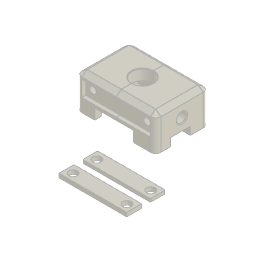
Obal_kamera (Autodesk Fusion 360 design; units mm, degrees)
part number: 2026-04-14-16-43-13-347
part number: 2026-04-14-16-45-35-834
Autodesk Fusion 360 part; units mm, degrees
sketch "Sketch1" plane through (0, 0, 0) normal (0, 0, 1) x (1, 0, 0) in component "kamera_obal"
  line L0 (-15, 10) -> (15, 10)
  line L1 (15, 10) -> (15, -10)
  line L2 (15, -10) -> (-15, -10)
  line L3 (-15, -10) -> (-15, 10)
  line L4 (-15, 10) -> (15, -10) construction
  line L5 (15, 10) -> (-15, -10) construction
  dimension "d1" = 20
  dimension "d2" = 30
  constraint horizontal L0
  constraint perpendicular L0 L1
  constraint parallel L0 L2
  constraint parallel L1 L3
  constraint coincident L4 origin
  constraint coincident L5 origin
  measures "d1" distance of L0.end L1.end
  measures "d2" distance of L1.end L2.end
extrude "Extrude1" add sketch "Sketch1" along normal blind 11 makes body 1 in component "kamera_obal"
sketch "Sketch4" plane through (0, 0, 11) normal (0, 0, 1) x (-1, 0, 0) in component "kamera_obal"
  line L0 (15, 10) -> (-15, 10)
  line L1 (-15, 10) -> (-15, -10)
  line L2 (-15, -10) -> (15, -10)
  line L3 (15, -10) -> (15, 10)
  circle A0 centre (0, 0) radius 4
  circle A1 centre (0, 0) radius 5.5
  dimension "d11" = 8
  dimension "d12" = 1.5
  constraint coincident A0.centre A1.centre
  measures "d11" diameter of A0
sketch "Sketch5" plane through (0, 0, 0) normal (0, 0, -1) x (1, 0, 0) in component "kamera_obal"
  line L0 (15, 10) -> (-15, 10)
  line L1 (-15, 10) -> (-15, -10)
  line L2 (-15, -10) -> (15, -10)
  line L3 (15, -10) -> (15, 10)
  line L4 (-4, 4) -> (4, 4) construction
  line L5 (4, 4) -> (4, -4) construction
  line L6 (4, -4) -> (-4, -4) construction
  line L7 (-4, -4) -> (-4, 4) construction
  line L8 (-4, 4) -> (4, -4) construction
  line L9 (4, 4) -> (-4, -4) construction
  line L10 (-4, 4) -> (-4, 7.4) construction
  line L11 (-4, 4) -> (-8, 4) construction
  line L12 (-4, -4) -> (-4, -6.3) construction
  line L13 (4, -4) -> (6.6, -4) construction
  line L14 (-4, -4) -> (-7.2, -4) construction
  line L15 (-7.2, -4) -> (-4, -4) construction
  line L16 (-4, -4) -> (-4, -6.3) construction
  line L17 (-4, -6.3) -> (-7.2, -6.3) construction
  line L18 (-7.2, -6.3) -> (-7.2, -4) construction
  line L19 (-4, -6.3) -> (6.5, -6.3) construction
  line L20 (6.6, -4) -> (4, -4) construction
  line L21 (4, -4) -> (4, -6.3) construction
  line L22 (4, -6.3) -> (6.6, -6.3) construction
  line L23 (6.6, -6.3) -> (6.6, -4) construction
  line L24 (-4, 7.4) -> (-8, 7.4) construction
  line L25 (-8, 7.4) -> (-8, 4) construction
  line L26 (-8, 4) -> (-4, 4) construction
  line L27 (-4, 4) -> (-4, 7.4) construction
  line L28 (6.6, -6.3) -> (-8.1, -6.3) construction
  line L29 (-8.1, -6.3) -> (-7.2, -6.3) construction
  line L30 (-7.2, -6.3) -> (6.1, -6.3) construction
  line L31 (6.1, -6.3) -> (6.6, -6.3) construction
  line L32 (6.6, -6.3) -> (-8.1, -6.3)
  line L33 (-8.1, -6.3) -> (-8.1, 7.5)
  line L34 (-8.1, 7.5) -> (6.6, 7.5)
  line L35 (6.6, 7.5) -> (6.6, -6.3)
  dimension "d13" = 8
  dimension "d14" = 8
  dimension "d15" = 4
  dimension "d17" = 2.3
  dimension "d18" = 2.6
  dimension "d143" = 4.1
  dimension "d144" = 3.5
  constraint horizontal L4
  constraint perpendicular L4 L5
  constraint parallel L4 L6
  constraint parallel L5 L7
  constraint coincident L8 origin
  constraint coincident L9 origin
  constraint perpendicular L4 L10
  constraint perpendicular L7 L11
  constraint perpendicular L6 L12
  constraint perpendicular L5 L13
  constraint perpendicular L12 L14
  constraint horizontal L15
  constraint vertical L16
  constraint horizontal L17
  constraint vertical L18
  constraint perpendicular L12 L19
  constraint horizontal L20
  constraint vertical L21
  constraint horizontal L22
  constraint vertical L23
  constraint coincident L19 L21.end
  constraint horizontal L24
  constraint vertical L25
  constraint horizontal L26
  constraint vertical L27
  constraint horizontal L28
  constraint horizontal L30
  constraint perpendicular L32 L33
  constraint parallel L32 L34
  constraint parallel L33 L35
  measures "d13" distance of L4.end L5.end
  measures "d14" distance of L5.end L6.end
  measures "d15" distance of L4.start L11.end
  measures "d17" distance of L6.end L12.end
  measures "d18" distance of L5.end L13.end
  measures "d143" distance of L7 L33
  measures "d144" distance of L4 L34
extrude "Extrude3" cut sketch "Sketch5" against normal blind 9 contours L32 L33 L34 L35 bodies 1 in component "kamera_obal"
extrude "Extrude4" add sketch "Sketch4" along normal blind 2.2 contours A1 bodies 1 in component "kamera_obal"
extrude "Extrude5" cut 1 faces at (-0.9485, -1.8197, 11) along direction (0, 0, -1) blind 2 on bodies 1 bodies 1 in component "kamera_obal"
extrude "Extrude25" add 1 faces at (-11.8333, 0, 11) along direction (0, 0, 1) blind 2.2 on bodies 1 bodies 1 in component "kamera_obal"
sketch "Sketch7" plane through (0, 10, 0) normal (0, 1, 0) x (-1, 0, 0) in component "kamera_obal"
  line L0 (-15, 13.2) -> (-15, 0)
  line L1 (-15, 0) -> (15, 0)
  line L2 (-6.6, 0) -> (-6.6, 9) construction
  line L3 (8.1, 0) -> (8.1, 9) construction
  line L4 (15, 0) -> (15, 13.2) construction
  line L5 (-6.6, 9) -> (8.1, 9) construction
  line L6 (-6.6, 0) -> (-6.6, 4)
  line L7 (-6.6, 4) -> (8.1, 4)
  line L8 (8.1, 4) -> (8.1, 0)
  line L9 (0, 4) -> (0, 5) construction
  line L10 (-13, 5) -> (13, 5) construction
  line L11 (-13, 5) -> (13, 5)
  line L12 (13, 5) -> (13, 11)
  line L13 (13, 11) -> (-13, 11)
  line L14 (-13, 11) -> (-13, 5)
  line L15 (15, 13.2) -> (-15, 13.2)
  point P0 (0, 5.5)
  dimension "d57" = 6
  dimension "d145" = 4
  dimension "d146" = 26
  dimension "d147" = 1
  constraint perpendicular L1 L6
  constraint perpendicular L2 L7
  constraint coincident L1 L3.start
  constraint perpendicular L1 L8
  constraint midpoint L9.end L10
  constraint horizontal L11
  constraint vertical L12
  constraint horizontal L13
  constraint vertical L14
  constraint coincident L3 L7.end
  constraint coincident L7 L9.start
  constraint horizontal L7.end L8.start
  constraint coincident L7.end L8.start
  constraint vertical L2.start L6.end
  constraint midpoint L9.end L11
  constraint vertical L9
  constraint vertical origin L9.start
  measures "d57" distance of L10.start L13.end
  measures "d145" distance of L7.end L3.start
  measures "d146" distance of L12.end L13.end
  measures "d147" distance of L7 L11
extrude "Extrude23" cut sketch "Sketch7" against normal blind 7 contours L1 L6 L7 L8 bodies 1 in component "kamera_obal"
extrude "Extrude8" cut sketch "Sketch7" against normal blind 1.5 contours L11 L12 L13 L14 bodies 1 in component "kamera_obal"
sketch "Sketch11" plane through (0, -10, 0) normal (0, -1, 0) x (1, 0, 0) in component "kamera_obal"
  line L0 (-15, 0) -> (15, 0)
  line L1 (15, 0) -> (15, 13.2)
  line L2 (-15, 13.2) -> (-15, 0)
  line L3 (13, 11) -> (-13, 11)
  line L4 (13, 5) -> (13, 11)
  line L5 (-13, 11) -> (-13, 5)
  line L6 (-13, 5) -> (13, 5)
  line L7 (6.6, 0) -> (6.6, 4)
  line L8 (6.6, 4) -> (-8.1, 4)
  line L9 (-8.1, 4) -> (-8.1, 0)
  line L10 (15, 13.2) -> (-15, 13.2)
extrude "Extrude24" cut sketch "Sketch11" against normal blind 7 contours L0 L7 L8 L9 bodies 1 in component "kamera_obal"
extrude "Extrude10" cut sketch "Sketch11" against normal blind 1.5 contours L3 L4 L5 L6 bodies 1 in component "kamera_obal"
sketch "Sketch9" plane through (15, 0, 0) normal (1, 0, 0) x (0, 1, 0) in component "kamera_obal"
  line L0 (-10, 0) -> (10, 0)
  line L1 (10, 0) -> (10, 13.2)
  line L2 (-10, 13.2) -> (-10, 0)
  circle A0 centre (0, 7.3632) radius 1.85
  line L3 (-10, 0) -> (-4.4, 0) construction
  line L4 (10, 0) -> (3.1, 0) construction
  line L5 (-4.4, 0) -> (-4.4, 3) construction
  line L6 (-4.4, 3) -> (3.1, 3)
  line L7 (3.1, 3) -> (3.1, 0)
  line L8 (3.1, 0) -> (-4.4, 0)
  line L9 (-4.4, 0) -> (-4.4, 3)
  line L10 (-10, 1.5263) -> (10, 13.2) construction
  line L11 (-10, 0) -> (10, 0)
  line L12 (10, 0) -> (10, 4)
  line L13 (10, 4) -> (6.3, 4)
  line L14 (6.3, 4) -> (6.3, 9)
  line L15 (6.3, 9) -> (-7.5, 9)
  line L16 (-7.5, 9) -> (-7.5, 4)
  line L17 (-7.5, 4) -> (-10, 4)
  line L18 (-10, 4) -> (-10, 0)
  line L19 (-7.5, 4) -> (-7.5, 0) construction
  line L20 (6.3, 4) -> (6.3, 0) construction
  line L21 (10, 13.2) -> (-10, 13.2)
  dimension "d41" = 3.7
  dimension "d66" = 3
  dimension "d154" = 3.1
  dimension "d155" = 4
  dimension "d156" = 3.2
  constraint coincident L0.start L2.end
  constraint perpendicular L2 L3
  constraint coincident L0.end L1.start
  constraint perpendicular L1 L4
  constraint perpendicular L3 L5
  constraint horizontal L6
  constraint vertical L7
  constraint horizontal L8
  constraint vertical L9
  constraint coincident L2 L10.start
  constraint coincident L1.end L10.end
  constraint midpoint A0.centre L10
  constraint coincident L16.end L17.start
  constraint coincident L11 L19.end
  constraint coincident L13.end L14.start
  constraint perpendicular L4 L20
  measures "d41" diameter of A0
  measures "d66" distance of L3.end L5.end
  measures "d154" distance of L5 L19
  measures "d155" distance of L13.end L20.end
  measures "d156" distance of L7 L20
sketch "Sketch10" plane through (-15, 0, 0) normal (-1, 0, 0) x (0, -1, 0) in component "kamera_obal"
  line L0 (-10, 0) -> (10, 0)
  line L1 (10, 0) -> (10, 13.2)
  line L2 (-10, 13.2) -> (-10, 0)
  circle A0 centre (0, 7.3632) radius 1.85
  line L3 (3, 3) -> (7.5, 3)
  line L4 (7.5, 3) -> (7.5, 0)
  line L5 (-10, 0) -> (10, 0)
  line L6 (10, 0) -> (10, 4)
  line L7 (10, 4) -> (7.5, 4)
  line L8 (7.5, 4) -> (7.5, 9)
  line L9 (7.5, 9) -> (-6.3, 9)
  line L10 (-6.3, 9) -> (-6.3, 4)
  line L11 (-6.3, 4) -> (-10, 4)
  line L12 (-10, 4) -> (-10, 0)
  line L13 (3, 3) -> (3, 0)
  line L14 (10, 13.2) -> (-10, 13.2)
  dimension "d152" = 4.5
  dimension "d153" = 3
  constraint horizontal L3
  constraint vertical L4
  constraint horizontal L0.end L4.end
  constraint coincident L0 L13.end
  constraint perpendicular L0 L13
  constraint vertical L3.end L7.end
  measures "d152" distance of L3.start L3.end
  measures "d153" distance of L3.end L4.end
extrude "Extrude12" cut sketch "Sketch9" against normal blind 4.7 contours A0 L15 | A0 L15 bodies 1 in component "kamera_obal"
extrude "Extrude13" cut sketch "Sketch9" against normal blind 15 contours L0 L6 L7 L8 L9 L11 bodies 1 in component "kamera_obal"
extrude "Extrude14" cut sketch "Sketch10" against normal blind 4.7 contours A0 L9 | A0 L9 bodies 1 in component "kamera_obal"
extrude "Extrude15" cut sketch "Sketch10" against normal blind 15 contours L0 L3 L4 L5 L13 bodies 1 in component "kamera_obal"
ref_plane "WorkPlane2" through (0, 0, 0) normal (1, 0, 0) x (0, 1, 0) in component "kamera_obal"
ref_plane "WorkPlane5" through (0, 8.5, 5.5) normal (0, 1, 0) x (-1, 0, 0) in component "kamera_obal"
sketch "Sketch14" plane through (0, 8.5, 0) normal (0, 1, 0) x (1, 0, 0) in component "kamera_obal"
  line L0 (6.6, -4) -> (6.6, -9)
  line L1 (-8.1, -4) -> (-8.1, -9)
  line L2 (13, -11) -> (-13, -11) construction
  line L3 (13, -5) -> (13, -11) construction
  line L4 (-13, -5) -> (13, -5) construction
  line L5 (-13, -11) -> (-13, -5) construction
  line L6 (6.6, -5) -> (6.6, -5.8) construction
  line L7 (6.6, -5.8) -> (12.5, -5.8) construction
  line L8 (8.05, -9.2) -> (8.05, -10) construction
  line L9 (8.05, -9.2) -> (13.95, -9.2) construction
  line L10 (8.05, -9.2) -> (9.05, -9.2) construction
  line L11 (9.05, -9.2) -> (11.45, -9.2) construction
  line L12 (11.45, -9.2) -> (11.45, -6.8) construction
  line L13 (11.45, -6.8) -> (9.05, -6.8) construction
  line L14 (9.05, -6.8) -> (9.05, -9.2) construction
  line L15 (11.45, -6.8) -> (9.05, -9.2) construction
  circle A0 centre (10.25, -8) radius 1.25
  line L16 (-8.1, -5) -> (-8.1, -5.8) construction
  line L17 (-8.1, -9) -> (-8.1, -9.2) construction
  line L18 (-9.05, -9.2) -> (-11.45, -9.2) construction
  line L19 (-9.05, -9.2) -> (-9.05, -6.8) construction
  line L20 (-9.05, -6.8) -> (-11.45, -9.2) construction
  circle A1 centre (-10.25, -8) radius 1.25
  line L21 (-8.1, -3) -> (-8.1, 0)
  dimension "d96" = 0.8
  dimension "d97" = 5.9
  dimension "d99" = 0.8
  dimension "d100" = 5.9
  dimension "d101" = 1
  dimension "d102" = 2.4
  dimension "d103" = 2.4
  dimension "d104" = 2.5
  dimension "d108" = 2.4
  dimension "d109" = 2.4
  dimension "d110" = 2.5
  dimension "d161" = 1.8
  dimension "d164" = 1.8
  dimension "d166" = 2.75
  dimension "d169" = 2.75
  constraint coincident L4 L6.start
  constraint coincident L0 L6.start
  constraint perpendicular L4 L6
  constraint perpendicular L3 L7
  constraint perpendicular L2 L8
  constraint perpendicular L3 L9
  constraint perpendicular L8 L10
  constraint horizontal L11
  constraint vertical L12
  constraint horizontal L13
  constraint vertical L14
  constraint midpoint L15 A0.centre
  constraint coincident L4 L16.start
  constraint coincident L1 L16.start
  constraint perpendicular L4 L16
  constraint coincident L1.end L17.start
  constraint perpendicular L2 L17
  constraint perpendicular L18 L19
  constraint midpoint L20 A1.centre
  constraint parallel L2 L18
  measures "d96" distance of L6.start L6.end
  measures "d97" distance of L6.end L7.end
  measures "d99" distance of L8.start L8.end
  measures "d100" distance of L8.start L9.end
  measures "d101" distance of L8.start L10.end
  measures "d102" distance of L10.end L13.end
  measures "d103" distance of L10.end L11.end
  measures "d104" diameter of A0
  measures "d108" distance of L18.start L18.end
  measures "d109" distance of L18.start L19.end
  measures "d110" diameter of A1
  measures "d161" distance of L4 L13
  measures "d164" distance of L2 L18
  measures "d166" distance of L5 A1.centre
  measures "d169" distance of L3 A0.centre
extrude "Extrude19" cut sketch "Sketch14" against normal blind 5 contours A0 bodies 1 in component "kamera_obal"
extrude "Extrude20" cut sketch "Sketch14" against normal blind 5 contours A1 bodies 1 in component "kamera_obal"
ref_plane "WorkPlane6" through (0, -8.5, 8) normal (0, -1, 0) x (0, 0, -1) in component "kamera_obal"
sketch "Sketch15" plane through (0, -8.5, 0) normal (0, -1, 0) x (-1, 0, 0) in component "kamera_obal"
  circle A0 centre (10.25, -8) radius 1.25
  circle A1 centre (-10.25, -8) radius 1.25
extrude "Extrude21" cut sketch "Sketch15" against normal blind 5 contours A0 bodies 1 in component "kamera_obal"
extrude "Extrude22" cut sketch "Sketch15" against normal blind 5 contours A1 bodies 1 in component "kamera_obal"
fillet "Fillet1" radius 2 4 edges at (15, 10, 5.5) (-15, 10, 5.5) (-15, -10, 5.5) (15, -10, 5.5) on bodies 1 in component "kamera_obal"
chamfer "Chamfer2" distance 2 distance2 1.5 8 edges at (0, -10, 13.2) (14.4142, -9.4142, 13.2) (15, 0, 13.2) (14.4142, 9.4142, 13.2) (0, 10, 13.2) (-14.4142, 9.4142, 13.2) (-15, 0, 13.2) (-14.4142, -9.4142, 13.2) measured on face at (-11.3333, 0, 13.2) measured on face at (13.0955, -9.9977, 8.8) measured on face at (-11.3333, 0, 13.2) measured on face at (14.7321, 9.0002, 8.8) measured on face at (-11.3333, 0, 13.2) measured on face at (-14.9977, 8.0955, 4.4) measured on face at (-11.3333, 0, 13.2) measured on face at (-13.0955, -9.9977, 4.4) on bodies 1 in component "kamera_obal"
sketch "Sketch2" plane through (0, 0, 0) normal (0, 0, 1) x (1, 0, 0)
  line L0 (4, -21) -> (29.7, -21)
  line L1 (29.7, -21) -> (29.7, -26.7)
  line L2 (29.7, -26.7) -> (4, -26.7)
  line L3 (4, -26.7) -> (4, -21)
  dimension "d124" = 5.7
  dimension "d125" = 25.7
  constraint horizontal L0
  constraint vertical L1
  constraint horizontal L2
  constraint vertical L3
  measures "d124" distance of L0.start L2.end
  measures "d125" distance of L0.start L0.end
extrude "Extrude1'" add sketch "Sketch2" along normal blind 1.5 separate body makes body 2
sketch "Sketch4 (2)" plane through (0, 0, 1.5) normal (0, 0, 1) x (-1, 0, 0)
  line L0 (-4, 26.7) -> (-29.7, 26.7)
  line L1 (-29.7, 26.7) -> (-29.7, 21)
  line L2 (-29.7, 21) -> (-4, 21)
  line L3 (-4, 21) -> (-4, 26.7)
  line L4 (-7.8185, 26.8595) -> (-7.8654, 25.2102) construction
  line L5 (-7.8654, 25.2102) -> (-5.4664, 25.142) construction
  line L6 (-7.8654, 25.2102) -> (-7.9336, 22.8112) construction
  line L7 (-5.4664, 25.142) -> (-7.9336, 22.8112) construction
  circle A0 centre (-6.7, 23.9766) radius 1.6
  line L8 (-25.793, 26.7352) -> (-25.7977, 25.0852) construction
  line L9 (-25.7977, 25.0852) -> (-25.8023, 22.6853) construction
  line L10 (-25.7977, 25.0852) -> (-28.1977, 25.0898) construction
  line L11 (-25.8023, 22.6853) -> (-28.1977, 25.0898) construction
  circle A1 centre (-27, 23.8875) radius 1.6
  dimension "d129" = 1.65
  dimension "d130" = 2.4
  dimension "d131" = 2.4
  dimension "d132" = 3.2
  dimension "d134" = 1.65
  dimension "d135" = 2.4
  dimension "d136" = 2.4
  dimension "d137" = 3.2
  dimension "d167" = 2.7
  dimension "d168" = 2.7
  constraint perpendicular L4 L5
  constraint perpendicular L5 L6
  constraint midpoint L7 A0.centre
  constraint perpendicular L9 L10
  constraint midpoint L11 A1.centre
  measures "d129" distance of L4.start L4.end
  measures "d130" distance of L4.end L5.end
  measures "d131" distance of L4.end L6.end
  measures "d132" diameter of A0
  measures "d134" distance of L8.start L8.end
  measures "d135" distance of L8.end L9.end
  measures "d136" distance of L8.end L10.end
  measures "d137" diameter of A1
  measures "d167" distance of L1 A1.centre
  measures "d168" distance of L3 A0.centre
extrude "Extrude2" cut sketch "Sketch4 (2)" against normal blind 1.5 contours A0 bodies 2
extrude "Extrude3'" cut sketch "Sketch4 (2)" against normal blind 1.5 contours A1 bodies 2
copy_body "CopyPasteBodies2" bodies 2 makes body 3
move_body "Move1" bodies 3 to x (1, 0, 0) y (0, 1, 0) z (0, 0, 1) at (0, -9, 0)
chamfer "Chamfer3" distance 0.2 angle 45 2 edges at (3.7293, 1.4465, 9) (3.7293, -1.4465, 13.2) on bodies 1 in component "kamera_obal"
chamfer "Chamfer4" distance 0.3 angle 45 2 edges at (15, -1.7248, 8.0321) (-15, 1.7248, 8.0321) on bodies 1 in component "kamera_obal"
chamfer "Chamfer1" distance 0.3 angle 45 8 edges at (29.7, -21, 0.75) (29.7, -26.7, 0.75) (16.85, -26.7, 0) (4, -26.7, 0.75) (4, -23.85, 0) (4, -21, 0.75) (16.85, -21, 0) (29.7, -23.85, 0) on bodies 2
split "Split1" by plane through (0, 0, 0) normal (1, 0, 0) bodies 1 makes body 4 at (10.0628, -0.1046, 13.2) in component "kamera_obal"
component "kamera_obal" placed x (1, 0, 0) y (0, 1, 0) z (0, 0, 1) at (0, 0, 0)
equation "d18 = 2.5 mm + 0.1 mm"
equation "d22 = 4.2 mm - 2 mm"
equation "vlozkaprumer = 4.1 mm"
equation "prumer_sroubu = 3 mm"
equation "d102 = prumer_sroubu - 0.2 * prumer_sroubu"
equation "d103 = prumer_sroubu - 0.2 * prumer_sroubu"
equation "d108 = prumer_sroubu - 0.2 * prumer_sroubu"
equation "d109 = prumer_sroubu - 0.2 * prumer_sroubu"
equation "d113 = -6.5 mm + 1.5 mm"
equation "d115 = -6.5 mm + 1.5 mm"
equation "d118 = -6.5 mm + 1.5 mm"
equation "d120 = -6.5 mm + 1.5 mm"
equation "d124 = 6 mm - 0.3 mm"
equation "d125 = 26 mm - 0.3 mm"
equation "d129 = 1.8 mm - 0.15 mm"
equation "d130 = prumer_sroubu - 0.2 * prumer_sroubu"
equation "d131 = prumer_sroubu - 0.2 * prumer_sroubu"
equation "d134 = 1.8 mm - 0.15 mm"
equation "d135 = prumer_sroubu - 0.2 * prumer_sroubu"
equation "d136 = prumer_sroubu - 0.2 * prumer_sroubu"
equation "d143 = 4 mm + 0.1 mm"
equation "d144 = 3.4 mm + 0.1 mm"
equation "d166 = 1.5 mm + d110 / 2"
equation "d169 = 1.5 mm + d104 / 2"
